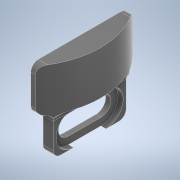
# Autodesk Inventor part: yystop
Saved by Autodesk Inventor 2022 (Build 260153000, 153)
## iProperties
Created: 2022-07-18
Part Number: yystop
Material: Genérico
Document SubType Name: Modeling
Designer: JK
Density: 1 g/cm^3
Appearance: Suave - Negro
Author: JK
Autodesk Inventor part; units mm, degrees
ref_plane "YZ Plane" through (0, 0, 0) normal (1, 0, 0) x (0, 1, 0)
ref_plane "XZ Plane" through (0, 0, 0) normal (0, 1, 0) x (-1, 0, 0)
ref_plane "XY Plane" through (0, 0, 0) normal (0, 0, 1) x (1, 0, 0)
sketch "Boceto1" plane through (0, 0, 0) normal (0, 1, 0) x (-1, 0, 0)
  line L0 (-14.8958, 21.4303) -> (7.8042, 21.4303)
  line L1 (7.8042, 21.4303) -> (7.8042, -5.2697)
  line L2 (7.8042, -5.2697) -> (-14.8958, -5.2697)
  line L3 (-14.8958, -5.2697) -> (-14.8958, 21.4303)
  line L4 (-14.8958, 21.4303) -> (7.8042, -5.2697) construction
  line L5 (7.8042, 21.4303) -> (-14.8958, -5.2697) construction
  arc A0 (-14.8958, 21.4303) -> (-14.8958, -5.2697) centre (2.3487, 8.0803) ccw
  line L6 (7.8042, 15.4612) -> (7.8042, 21.4303)
  line L7 (-13.6958, 18.2303) -> (6.6042, 18.2303)
  line L8 (6.6042, 18.2303) -> (6.6042, -2.0697)
  line L9 (6.6042, -2.0697) -> (-13.6958, -2.0697)
  line L10 (-13.6958, -2.0697) -> (-13.6958, 18.2303)
  line L11 (-13.6958, 18.2303) -> (6.6042, -2.0697) construction
  line L12 (6.6042, 18.2303) -> (-13.6958, -2.0697) construction
  line L13 (7.8042, 21.4303) -> (11.6042, 21.4303)
  line L14 (11.6042, 21.4303) -> (11.6042, -5.2697)
  line L15 (11.6042, -5.2697) -> (7.8042, -5.2697)
  line L16 (7.8042, -5.2697) -> (7.8042, 21.4303)
  line L17 (7.8042, 21.4303) -> (6.6042, 21.4303)
  line L18 (6.6042, 21.4303) -> (6.6042, -5.2697)
  line L19 (6.6042, -5.2697) -> (7.8042, -5.2697)
  line L20 (7.8042, -5.2697) -> (7.8042, 21.4303)
  line L21 (11.6042, -5.2697) -> (6.6042, -5.2697)
  line L22 (6.6042, -5.2697) -> (6.6042, -2.0697)
  line L23 (6.6042, -2.0697) -> (11.6042, -2.0697)
  line L24 (11.6042, -2.0697) -> (11.6042, -5.2697)
  line L25 (11.6042, 21.4303) -> (6.6042, 21.4303)
  line L26 (6.6042, 21.4303) -> (6.6042, 18.2303)
  line L27 (6.6042, 18.2303) -> (11.6042, 18.2303)
  line L28 (11.6042, 18.2303) -> (11.6042, 21.4303)
  line L29 (-14.8958, 21.4303) -> (-13.6958, 21.4303)
  line L30 (-13.6958, 21.4303) -> (-13.6958, -5.2697)
  line L31 (-13.6958, -5.2697) -> (-14.8958, -5.2697)
  line L32 (-14.8958, -5.2697) -> (-14.8958, 21.4303)
  point P0 (-3.5458, 8.0803)
  point P1 (6.6042, -2.0697)
  point P2 (6.6042, 18.2303)
  point P3 (6.6042, 18.2303)
  point P4 (6.6042, -2.0697)
  point P5 (-13.6958, -2.0697)
  dimension "d4" = 20.3
  dimension "d5" = 3.2
  dimension "d6" = 1.2
  dimension "d7" = 20.3
  dimension "d14" = 5
  constraints: 66 end point, 14 parallel, 7 horizontal, 7 perpendicular, 4 midpoint, 4 point on line, 2 point on circle, 1 centre point
  measures "d4" distance of L7.end L8.end
  measures "d5" distance between parallel lines of L7 L0
  measures "d6" distance between parallel lines of L10 L3
  measures "d7" distance of L7.start L7.end
  measures "d14" distance between parallel lines of L14 L18
extrude "Extrusión1" add sketch "Boceto1" along normal blind 12 contours L0 L30 L10 L2 L3 | L3 A0
sketch "Boceto3" plane through (0, 0, 0) normal (0, -1, 0) x (1, 0, 0)
  line L0 (10.8958, -1.9197) -> (16.4958, -1.9197)
  line L1 (16.4958, -1.9197) -> (16.4958, 18.0803)
  line L2 (16.4958, 18.0803) -> (10.8958, 18.0803)
  line L3 (10.8958, 18.0803) -> (10.8958, -1.9197)
  line L4 (13.6958, -5.2697) -> (13.6958, 21.4303) projected
  line L5 (10.8958, -1.9197) -> (16.4958, 18.0803) construction
  line L6 (16.4958, -1.9197) -> (10.8958, 18.0803) construction
  point P0 (0, 0)
  point P1 (13.6958, 8.0803)
  point P2 (13.6958, 18.0803)
  point P3 (13.6958, -1.9197)
  dimension "d18" = 20
  dimension "d19" = 2.8
  constraints: 12 end point, 3 midpoint, 2 parallel, 1 horizontal, 1 perpendicular
  measures "d18" distance of L2.end L0.start
  measures "d19" distance between parallel lines of L4 L1
extrude "Extrusión3" add sketch "Boceto3" along normal blind 11 contours L4 L2 L1 L0
fillet "Empalme2" radius 2 9 edges at (15.0958, 0, 18.0803) (15.0958, -11, 18.0803) (15.0958, -11, -1.9197) (15.0958, 0, -1.9197) (14.2958, 0, -5.2697) (14.2958, 12, -5.2697) (14.2958, 0, 21.4303) (14.2958, 12, 21.4303) (16.4958, 0, 8.0803)
sketch "Boceto4" plane through (16.4958, -9, -1.9197) normal (1, 0, 0) x (0, 0, -1)
  circle A0 centre (-14.5, 2.7) radius 2.7
  circle A1 centre (-5.5, 2.7) radius 2.7
  line L0 (-14.5, 5.4) -> (-5.5, 5.4)
  line L1 (-5.5, 5.4) -> (-5.5, 0)
  line L2 (-5.5, 0) -> (-14.5, 0)
  line L3 (-14.5, 0) -> (-14.5, 5.4)
  line L4 (-20, 7) -> (-20, 0) projected
  line L5 (0, 7) -> (0, 0) projected
  line L6 (-2, -2) -> (-18, -2) projected
  point P0 (-1.9197, 9)
  point P1 (-5.5, 0)
  point P2 (-5.5, 5.4)
  dimension "d23" = 5.4
  dimension "d24" = 5.5
  dimension "d25" = 5.5
  dimension "d26" = 2
  constraints: 8 end point, 4 tangent, 2 centre point, 2 midpoint, 2 parallel, 1 horizontal, 1 perpendicular
  measures "d23" diameter of A0
  measures "d24" distance from line of L4 A0.centre
  measures "d25" distance from line of L5 A1.centre
  measures "d26" distance between parallel lines of L2 L6
extrude "Extrusión4" cut sketch "Boceto4" against normal through all
sketch "Boceto5" plane through (16.4958, -9, -1.9197) normal (1, 0, 0) x (0, 0, -1)
  arc A0 (-5.5, 0) -> (-5.5, 5.4) centre (-5.5, 2.7) ccw projected
  line L0 (-5.5, 0) -> (-14.5, 0) projected
  arc A1 (-14.5, 5.4) -> (-14.5, 0) centre (-14.5, 2.7) ccw projected
  line L1 (-14.5, 5.4) -> (-5.5, 5.4) projected
  arc A2 (-2, -2) -> (0, 0) centre (-2, 0) ccw projected
  line L2 (0, 7) -> (0, 0) projected
  line L3 (-20, 7) -> (0, 7) projected
  line L4 (-20, 7) -> (-20, 0) projected
  arc A3 (-20, 0) -> (-18, -2) centre (-18, 0) ccw projected
  line L5 (-2, -2) -> (-18, -2) projected
  arc A4 (-5.5, -2) -> (-5.5, 7.4) centre (-5.5, 2.7) ccw
  line L6 (-5.5, -2) -> (-14.5, -2)
  arc A5 (-14.5, 7.4) -> (-14.5, -2) centre (-14.5, 2.7) ccw
  line L7 (-14.5, 7.4) -> (-5.5, 7.4)
  point P0 (-1.9197, 9)
  point P1 (-16.3974, 7)
  point P2 (-14.5, -2)
  point P3 (-5.5, -2)
  point P4 (-3.6026, 7)
  dimension "d29" = 2
  constraints: 4 end point, 4 point on circle, 2 centre point, 3 other
  measures "d29" distance between parallel lines of L1 L7
extrude "Extrusión5" cut sketch "Boceto5" along normal blind 9.65 and the other way blind 1.4 contours L5 A5 L3 A4
sketch "Boceto2" plane through (-6.6042, 0, 21.4303) normal (0, 0, 1) x (1, 0, 0)
  circle A0 centre (2.3, 6) radius 2.7
  line L0 (-5, 0) -> (21.5, 0) projected
  circle A1 centre (10.3, 6) radius 2.7
  line L1 (2.3, 3.3) -> (10.3, 3.3)
  line L2 (10.3, 3.3) -> (10.3, 8.7)
  line L3 (10.3, 8.7) -> (2.3, 8.7)
  line L4 (2.3, 8.7) -> (2.3, 3.3)
  point P0 (6.6042, 0)
  point P1 (20.3, 0)
  dimension "d10" = 5.4
  dimension "d11" = 6
  dimension "d12" = 10
  dimension "d13" = 8
  constraints: 8 end point, 2 horizontal, 2 parallel, 2 tangent, 1 centre point, 1 perpendicular, 1 vertical alignment, 3 other
  measures "d11" distance from line of L0 point (2.3, 6)
  measures "d12" horizontal distance of point (20.3, 0) A1.centre
  measures "d13" distance of L1.start L1.end
